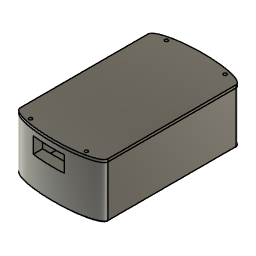
Bateria (Autodesk Fusion 360 design; units mm, degrees)
Autodesk Fusion 360 part; units mm, degrees
sketch "Boceto1" plane through (0, 0, 0) normal (0, 0, 1) x (1, 0, 0)
  line L0 (15.5, -24) -> (-15.5, -24)
  line L1 (-15.5, -24) -> (-15.5, 24)
  line L2 (-15.5, 24) -> (15.5, 24)
  line L3 (15.5, 24) -> (15.5, -24)
  line L4 (15.5, -24) -> (-15.5, 24) construction
  line L5 (-15.5, -24) -> (15.5, 24) construction
  line L6 (-16.5, -24) -> (-16.5, 24)
  line L7 (16.5, 24) -> (16.5, -24)
  line L8 (16.5, -25) -> (-16.2747, 24.6587) construction
  line L9 (-16.5, -25) -> (16.2747, 24.6587) construction
  ellipse E0 centre (0, 24) end of major axis (16.5, 24) minor radius 4 (16.5, 24) -> (-16.5, 24) ccw
  ellipse E1 centre (0, -24) end of major axis (16.5, -24) minor radius 4 (-16.5, -24) -> (16.5, -24) ccw
  dimension "d1" = 31
  dimension "d2" = 48
  dimension "d6" = 8
  constraint horizontal L0
  constraint perpendicular L0 L1
  constraint parallel L0 L2
  constraint parallel L1 L3
  constraint coincident L4 origin
  constraint coincident L5 origin
  constraint parallel L6 L7
  constraint coincident L8 origin
  constraint coincident L9 origin
  constraint midpoint L0 E1.centre
  measures "d1" distance of L1.end L2.end
  measures "d2" distance of L0.end L1.end
extrude "Extruir1" add sketch "Boceto1" against normal blind 1 contours L0 L1 L2 L3 | L6 L7 E0 E1 makes body 1
extrude "Extruir2" add sketch "Boceto1" along normal blind 0.8 from surface at 30 separate body contours L0 L1 L2 L3 makes body 2
extrude "Extruir3" add sketch "Boceto1" along normal blind 18.5 bodies 1
extrude "Extruir4" add sketch "Boceto1" along normal blind 1 from surface at 18.5 separate body contours L0 L1 L2 L3 | L6 L7 E0 E1 makes body 3
ref_plane "PlanoDeObra1" through (0, -28, 0) normal (0, 1, 0) x (0, 0, 1)
sketch "Boceto4" plane through (0, -28, 0) normal (0, 1, 0) x (1, 0, 0)
  line L0 (-16.5, -18.5) -> (-16.5, 1)
  line L1 (16.5, 1) -> (-16.5, 1)
  line L2 (16.5, 1) -> (16.5, -18.5)
  line L3 (-16.5, -18.5) -> (16.5, -18.5)
  line L4 (-16.5, -18.5) -> (16.5, -18.5)
  line L5 (16.5, -18.5) -> (16.5, -19.5)
  line L6 (-16.5, -19.5) -> (16.5, -19.5)
  line L7 (-16.5, -19.5) -> (-16.5, -18.5)
  line L8 (0, -19.5) -> (-14, -19.5) construction
  line L9 (-14, -19.5) -> (-14, -12.5) construction
  line L10 (-14, -12.5) -> (0, -12.5) construction
  line L11 (0, -19.5) -> (0, -12.5) construction
  line L12 (-14, -12.5) -> (-14, -10.5) construction
  line L13 (-14, -10.5) -> (-8, -10.5) construction
  line L14 (-8, -10.5) -> (4, -10.5)
  line L15 (4, -10.5) -> (4, -16.5)
  line L16 (4, -16.5) -> (-8, -16.5)
  line L17 (-8, -16.5) -> (-8, -10.5)
  dimension "d18" = 14
  dimension "d19" = 7
  dimension "d20" = 14
  dimension "d40" = 2
  dimension "d41" = 6
  dimension "d43" = 12
  dimension "d44" = 6
  constraint midpoint L6 L8.start
  constraint parallel L6 L8
  constraint perpendicular L3 L9
  constraint perpendicular L9 L10
  constraint perpendicular L10 L12
  constraint perpendicular L12 L13
  constraint horizontal L14
  constraint vertical L15
  constraint horizontal L16
  constraint vertical L17
  measures "d18" distance of L8.start L8.end
  measures "d19" distance of L8.end L9.end
  measures "d20" distance of L9.end L10.end
  measures "d40" distance of L9.end L12.end
  measures "d41" distance of L12.end L13.end
  measures "d43" distance of L13.end L14.end
  measures "d44" distance of L13.end L16.end
extrude "Extruir5" cut sketch "Boceto4" along normal blind 6 contours L14 L15 L16 L17 bodies 1
fillet "Empalme1" radius 0.5 4 edges at (-16.5, 0, -1) (0, 28, -1) (16.5, 0, -1) (0, -28, -1) on bodies 1
sketch "Boceto6" plane through (0, 0, 19.5) normal (0, 0, 1) x (-1, 0, 0)
  line L0 (-16.5, 24) -> (-16.5, -24)
  ellipse E0 centre (0, -24) end of major axis (-16.5, -24) minor radius 4 (-16.5, -24) -> (16.5, -24) ccw
  line L1 (16.5, -24) -> (16.5, 24)
  ellipse E1 centre (0, 24) end of major axis (-16.5, 24) minor radius 4 (16.5, 24) -> (-16.5, 24) ccw
  line L2 (15.5, -24) -> (-15.5, -24)
  line L3 (-15.5, 24) -> (15.5, 24)
  line L4 (0, -24) -> (0, -28) construction
  line L5 (0, -25.073) -> (11, -25.073) construction
  line L6 (0, -25.073) -> (-11, -25.073) construction
  line L7 (-11, -25.073) -> (-11, -24) construction
  line L8 (11, -25.073) -> (11, -24) construction
  line L9 (-11, -24) -> (-11, -25.4)
  circle A0 centre (-11, -25.4) radius 0.6
  line L10 (11, -24) -> (11, -25.4) construction
  circle A1 centre (11, -25.4) radius 0.6
  line L11 (0, 24) -> (-10, 24) construction
  line L12 (-10, 24) -> (-10, 27.1817) construction
  line L13 (0, 24) -> (11, 24) construction
  line L14 (11, 24) -> (11, 26.9814) construction
  circle A2 centre (11, 25.4907) radius 0.6
  circle A3 centre (-10, 25.5908) radius 0.6
  dimension "d31" = 11
  dimension "d32" = 11
  dimension "d34" = 1.4
  dimension "d35" = 1.2
  dimension "d36" = 1.4
  dimension "d37" = 1.2
  dimension "d46" = 10
  dimension "d47" = 11
  dimension "d48" = 1.2
  dimension "d49" = 1.2
  constraint coincident E0.centre L4.start
  constraint coincident E0 L4.end
  constraint perpendicular L2 L4
  constraint coincident L4 L5.start
  constraint perpendicular L4 L5
  constraint perpendicular L4 L6
  constraint coincident L2 L7.end
  constraint perpendicular L2 L7
  constraint coincident L2 L8.end
  constraint perpendicular L2 L8
  constraint perpendicular L6 L9
  constraint coincident L9.end A0.centre
  constraint perpendicular L5 L10
  constraint coincident L10.end A1.centre
  constraint coincident E1.centre L11.start
  constraint coincident E1 L12.end
  constraint perpendicular L3 L12
  constraint parallel L3 L13
  constraint coincident E1 L14.end
  constraint perpendicular L13 L14
  constraint midpoint L14 A2.centre
  constraint midpoint L12 A3.centre
  measures "d31" distance of L5.start L5.end
  measures "d32" distance of L5.start L6.end
  measures "d34" distance of L7.end L9.end
  measures "d35" diameter of A0
  measures "d36" distance of L8.end L10.end
  measures "d37" diameter of A1
  measures "d46" distance of E1.centre L11.end
  measures "d47" distance of E1.centre L13.end
  measures "d48" diameter of A2
  measures "d49" diameter of A3
extrude "Extruir7" cut sketch "Boceto6" against normal blind 8 contours A0 | A1 | A2 | A3 bodies 1 3
hidden bodies 2
equation "d12 = 12 mm + 6.5 mm"
named bodies: "Bat_case", "Bat_prot", "Bat_tap"
